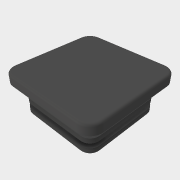
# Autodesk Inventor part: PWTR-0123
Saved by Autodesk Inventor 2021.1 (Build 251245000, 245)
## iProperties
Created: 2020-09-02
Part Number: PWTR-0123
Material: Rubber
Document SubType Name: Modeling
Designer: alid
Density: 0.93 g/cm^3
Appearance: Rubber - Black
Description: Arm End Cap
Author: alid
Revision Number: A
Autodesk Inventor part; units mm, degrees
ref_plane "YZ Plane" through (0, 0, 0) normal (1, 0, 0) x (0, 1, 0)
ref_plane "XZ Plane" through (0, 0, 0) normal (0, 1, 0) x (-1, 0, 0)
ref_plane "XY Plane" through (0, 0, 0) normal (0, 0, 1) x (1, 0, 0)
sketch "Sketch1" plane through (0, 0, 0) normal (0, 0, 1) x (1, 0, 0)
  line L0 (16, -16) -> (-16, -16)
  line L1 (-16, -16) -> (-16, 16)
  line L2 (-16, 16) -> (16, 16)
  line L3 (16, 16) -> (16, -16)
  line L4 (16, -16) -> (-16, 16) construction
  line L5 (-16, -16) -> (16, 16) construction
  line L6 (14, 14) -> (-14, 14)
  line L7 (-14, 14) -> (-14, -14)
  line L8 (-14, -14) -> (14, -14)
  line L9 (14, -14) -> (14, 14)
  line L10 (20, -20) -> (-20, -20)
  line L11 (-20, -20) -> (-20, 20)
  line L12 (-20, 20) -> (20, 20)
  line L13 (20, 20) -> (20, -20)
  line L14 (-11, 11) -> (11, 11)
  line L15 (11, 11) -> (11, -11)
  line L16 (11, -11) -> (-11, -11)
  line L17 (-11, -11) -> (-11, 11)
  point P0 (0, 0)
  dimension "d0" = 32
  dimension "d1" = 32
  dimension "d2" = 2
  dimension "d10" = 4
  dimension "d12" = 3
  constraints: 36 end point, 8 parallel, 4 perpendicular, 2 midpoint, 1 horizontal, 9 other
  measures "d0" distance of L1.end L2.end
  measures "d1" distance of L0.end L1.end
  measures "d2" distance between parallel lines of L2 L6
  measures "d10" distance between parallel lines of L3 L13
  measures "d12" distance between parallel lines of L6 L14
extrude "Extrusion1" add sketch "Sketch1" against normal blind 2 contours L9 L8 L7 L6 | L14 L15 L16 L17
extrude "Extrusion2" add sketch "Sketch1" against normal blind 2 from surface at -2 contours L0 L1 L2 L3 | L9 L8 L7 L6 | L14 L15 L16 L17
fillet "Fillet1" radius 4 8 edges at (-16, 16, -3) (16, 16, -3) (-16, -16, -3) (14, -14, -1) (-14, -14, -1) (-14, 14, -1) (14, 14, -1) (16, -16, -3)
pattern_linear "Rectangular Pattern1" count 3 spacing 4 along (0, 0, -1)
extrude "Extrusion3" add sketch "Sketch1" along normal blind 4 contours L0 L1 L2 L3 | L9 L8 L7 L6 | L10 L11 L12 L13 | L14 L15 L16 L17
fillet "Fillet2" radius 5 4 edges at (-20, 20, 2) (20, 20, 2) (-20, -20, 2) (20, -20, 2)
extrude "Extrusion4" cut sketch "Sketch1" against normal through all contours L14 L15 L16 L17
fillet "Fillet3" radius 1 8 edges at (0, 20, 4) (-18.5355, 18.5355, 4) (-20, 0, 4) (-18.5355, -18.5355, 4) (0, -20, 4) (18.5355, -18.5355, 4) (20, 0, 4) (18.5355, 18.5355, 4)
body "Solid1"
